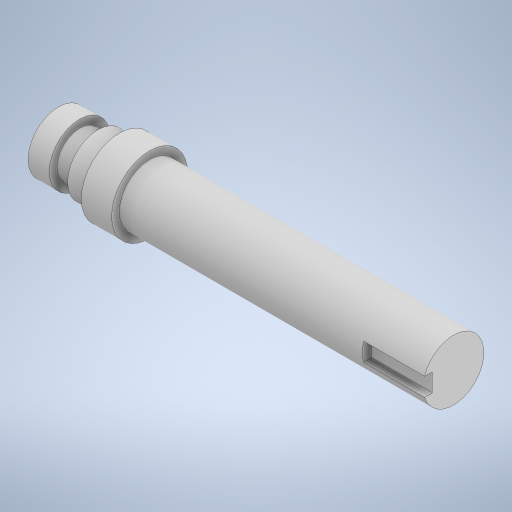
# Autodesk Inventor part: shaft
Saved by Autodesk Inventor 2024 (Build 280153000, 153)
## iProperties
Created: 2023-10-30
Part Number: shaft
Material: Generic
Document SubType Name: Modeling
Designer: Admin
Density: 1 g/cm^3
Appearance: Default
Author: Admin
Autodesk Inventor part; units mm, degrees
ref_plane "XZ Plane" through (0, 0, 0) normal (0, 1, 0) x (-1, 0, 0)
ref_plane "XY Plane" through (0, 0, 0) normal (0, 0, 1) x (1, 0, 0)
sketch "Sketch1" plane through (0, 0, 0) normal (1, 0, 0) x (0, 1, 0)
  circle A0 centre (0, 0) radius 12.5
  circle A1 centre (0, 0) radius 10
  dimension "d0" = 25
  dimension "d1" = 20
  constraints: 2 centre point, 2 coincident
  measures "d0" diameter of A0
  measures "d1" diameter of A1
extrude "Extrusion1" add sketch "Sketch1" against normal blind 130 contours A0 | A1
extrude "Extrusion2" cut sketch "Sketch1" against normal blind 100
sketch "Sketch3" plane through (-130, 0, 0) normal (-1, 0, 0) x (0, 0, 1)
  circle A0 centre (0, 0) radius 10 projected
  circle A1 centre (0, 0) radius 9.5
  circle A2 centre (0, 0) radius 12.5
  dimension "d7" = 19
  dimension "d19" = 25
  constraints: 2 centre point, 2 coincident
  measures "d7" diameter of A1
  measures "d19" diameter of A2
extrude "Extrusion3" cut sketch "Sketch3" against normal blind 20 contours A2
ref_plane "Work Plane2" through (-123, 0, 0) normal (1, 0, 0) x (0, 1, 0)
sketch "Sketch4" plane through (-123, 0, 0) normal (1, 0, 0) x (0, 1, 0)
  circle A0 centre (0, 0) radius 7.5
  circle A1 centre (0, 0) radius 10
  dimension "d11" = 15
  dimension "d20" = 20
  constraints: 2 centre point, 2 coincident
  measures "d11" diameter of A0
  measures "d20" diameter of A1
extrude "Extrusion4" cut sketch "Sketch4" along normal blind 6
sketch "Sketch5" plane through (0, 0, 0) normal (1, 0, 0) x (0, 0, -1)
  line L0 (-7, 3) -> (-9.5394, 3)
  line L1 (-7, 3) -> (-7, -3)
  line L2 (-7, -3) -> (-9.5394, -3)
  circle A0 centre (0, 0) radius 10 projected
  arc A1 (-9.5394, 3) -> (-9.5394, -3) centre (0, 0) ccw
  point P0 (-7, 0)
  dimension "d14" = 7
  dimension "d15" = 6
  dimension "d16" = 3
  constraints: 6 end point, 4 point on circle, 2 vertical alignment, 1 centre point, 1 coincident, 1 horizontal, 1 horizontal alignment, 1 perpendicular, 1 vertical
  measures "d14" distance of point (0, 0) point (-7, 0)
  measures "d15" distance of L0.start L1.end
  measures "d16" distance of point (-7, 0) L1.end
extrude "Extrusion5" cut sketch "Sketch5" against normal blind 20 contours L1 L2 A0 L0 picked at (-7.9828, -0.338)
body "Solid1"
